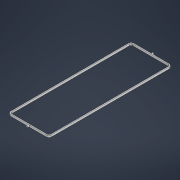
# Autodesk Inventor part: 30t_8.5_in
Saved by Autodesk Inventor 2021 (Build 250183000, 183)
## iProperties
Created: 2020-12-06
Part Number: 30t_8.5_in
Material: Generic
Document SubType Name: Modeling
Designer: Carlos Stewart
Density: 1 g/cm^3
Appearance: Default
Author: Carlos Stewart
Autodesk Inventor part; units mm, degrees
ref_plane "YZ Plane" through (0, 0, 0) normal (1, 0, 0) x (0, 1, 0)
ref_plane "XZ Plane" through (0, 0, 0) normal (0, 1, 0) x (-1, 0, 0)
ref_plane "XY Plane" through (0, 0, 0) normal (0, 0, 1) x (1, 0, 0)
sketch "Sketch1" plane through (0, 0, 0) normal (0, 1, 0) x (-1, 0, 0)
  line L0 (-3.175, 0) -> (-66.675, 0)
  line L1 (-69.85, -3.175) -> (-69.85, -213.3854)
  line L2 (-66.675, -216.5604) -> (-3.175, -216.5604)
  line L3 (0, -213.3854) -> (0, -3.175)
  arc A0 (0, -3.175) -> (-3.175, 0) centre (-3.175, -3.175) ccw
  arc A1 (-66.675, 0) -> (-69.85, -3.175) centre (-66.675, -3.175) ccw
  arc A2 (-69.85, -213.3854) -> (-66.675, -216.5604) centre (-66.675, -213.3854) ccw
  arc A3 (-3.175, -216.5604) -> (0, -213.3854) centre (-3.175, -213.3854) ccw
  line L4 (1.5875, -3.175) -> (1.5875, -213.3854)
  arc A4 (-3.175, -218.1479) -> (1.5875, -213.3854) centre (-3.175, -213.3854) ccw
  line L5 (-3.175, -218.1479) -> (-66.675, -218.1479)
  arc A5 (-71.4375, -213.3854) -> (-66.675, -218.1479) centre (-66.675, -213.3854) ccw
  line L6 (-71.4375, -213.3854) -> (-71.4375, -3.175)
  arc A6 (-66.675, 1.5875) -> (-71.4375, -3.175) centre (-66.675, -3.175) ccw
  line L7 (-66.675, 1.5875) -> (-3.175, 1.5875)
  arc A7 (1.5875, -3.175) -> (-3.175, 1.5875) centre (-3.175, -3.175) ccw
  point P0 (0, 0)
  point P1 (-69.85, -216.5604)
  point P2 (-69.85, 0)
  point P3 (0, -216.5604)
  dimension "d0" = 69.85
  dimension "d1" = 216.5604
  dimension "d2" = 3.175
  constraints: 16 end point, 16 point on circle, 8 centre point, 8 point on line, 8 tangent, 4 parallel, 3 equal radius, 2 perpendicular, 1 horizontal, 7 other
  measures "d0" distance of point (0, -216.56) point (-69.85, -216.56)
  measures "d1" distance of point (-69.85, -216.56) point (-69.85, 0)
  measures "d2" radius of A0
extrude "Extrusion2" add sketch "Sketch1" along normal blind 3.175
sketch "Sketch4" plane through (3.175, 0, 1.5875) normal (0, 0, 1) x (1, 0, 0)
  circle A0 centre (31.75, 1.5875) radius 1.5875
  line L0 (0, 0) -> (0, 3.175) projected
  line L1 (0, 0) -> (63.5, 0) projected
  point P0 (-3.175, 0)
  dimension "d11" = 3.175
  dimension "d12" = 31.75
  dimension "d13" = 1.5875
  constraints: 1 centre point
  measures "d11" diameter of A0
  measures "d12" distance from line of L0 A0.centre
  measures "d13" distance from line of L1 A0.centre
extrude "Extrusion3" add sketch "Sketch4" along normal blind 2.54
sketch "Sketch5" plane through (66.675, 0, -218.1479) normal (0, 0, -1) x (-1, 0, 0)
  arc A0 (31.75, 0) -> (31.75, 3.175) centre (31.75, 1.5875) ccw projected
  circle A1 centre (31.75, 1.5875) radius 1.5875
  point P0 (66.675, 0)
  point P1 (31.75, 3.175)
  point P2 (31.75, 0)
  constraints: 1 centre point, 1 coincident
extrude "Extrusion4" add sketch "Sketch5" along normal blind 2.54
body "Solid2"
